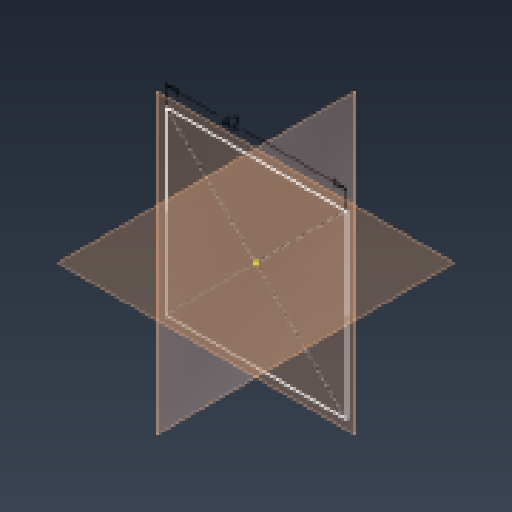
# Autodesk Inventor part: Крепление_мотора_V2
Saved by Autodesk Inventor 2023.2 (Build 272271030, 271C)
## iProperties
Created: 2025-12-26
Part Number: Крепление_мотора_V2
Material: Типовые
Document SubType Name: Modeling
Designer: Олег Коноваленко
Density: 1 g/cm^3
Appearance: По умолчанию
Author: Олег Коноваленко
Autodesk Inventor part; units mm, degrees
sketch "Эскиз1" plane through (0, 0, 0) normal (0, 0, 1) x (1, 0, 0)
  line L0 (21, -21) -> (-21, -21)
  line L1 (-21, -21) -> (-21, 21)
  line L2 (-21, 21) -> (21, 21)
  line L3 (21, 21) -> (21, -21)
  line L4 (21, -21) -> (-21, 21) construction
  line L5 (-21, -21) -> (21, 21) construction
  point P0 (0, 0)
  dimension "d0" = 42
  constraints: 12 end point, 2 midpoint, 2 parallel, 2 perpendicular, 1 horizontal
  measures "d0" distance of L1.end L2.end
extrude "Выдавливание1" add sketch "Эскиз1" along normal blind 12
sketch "Эскиз2" plane through (0, 0, 12) normal (0, 0, 1) x (1, 0, 0)
  circle A0 centre (0, 0) radius 11.6
  dimension "d3" = 23.2
  constraints: 1 centre point, 1 coincident
  measures "d3" diameter of A0
extrude "Выдавливание2" cut sketch "Эскиз2" against normal up to next
sketch "Эскиз3" plane through (0, 0, 12) normal (0, 0, 1) x (1, 0, 0)
  circle A0 centre (-15.5, 15.5) radius 1.35
  circle A1 centre (15.5, 15.5) radius 1.35
  circle A2 centre (-15.5, -15.5) radius 1.35
  circle A3 centre (15.5, -15.5) radius 1.35
  line L0 (-15.5, 15.5) -> (-15.5, -15.5) construction
  line L1 (-15.5, -15.5) -> (15.5, -15.5) construction
  line L2 (15.5, -15.5) -> (15.5, 15.5) construction
  line L3 (15.5, 15.5) -> (-15.5, 15.5) construction
  line L4 (-15.5, 15.5) -> (15.5, -15.5) construction
  line L5 (15.5, 15.5) -> (-15.5, -15.5) construction
  point P0 (0, 0)
  point P1 (0, 0)
  dimension "d6" = 2.7
  dimension "d7" = 31
  constraints: 12 end point, 4 centre point, 4 perpendicular, 3 equal radius, 1 coincident, 1 horizontal, 1 midpoint, 1 parallel, 1 point on line
  measures "d6" diameter of A0
  measures "d7" distance of L2.end L0.start
extrude "Выдавливание3" cut sketch "Эскиз3" against normal up to next
